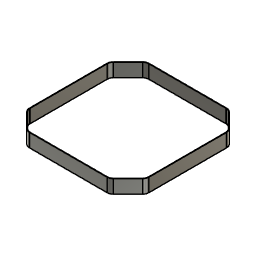
Drone Top Lid LED Face (Autodesk Fusion 360 design; units mm, degrees)
Autodesk Fusion 360 part; units mm, degrees
sketch "Sketch1" plane through (0, 0, 0) normal (0, 0, 1) x (1, 0, 0)
  line L0 (64.1079, 98.25) -> (-64.1079, 98.25)
  line L1 (-98.25, 64.1079) -> (-98.25, -64.1079)
  line L2 (-64.1079, -98.25) -> (64.1079, -98.25)
  line L3 (98.25, -64.1079) -> (98.25, 64.1079)
  line L4 (98.25, 98.25) -> (-98.25, -98.25) construction
  line L5 (-98.25, 98.25) -> (98.25, -98.25) construction
  line L6 (-95.3211, 71.1789) -> (-71.1789, 95.3211)
  arc A0 (-64.1079, 98.25) -> (-71.1789, 95.3211) centre (-64.1079, 88.25) ccw
  arc A1 (-95.3211, 71.1789) -> (-98.25, 64.1079) centre (-88.25, 64.1079) ccw
  line L7 (71.1789, 95.3211) -> (95.3211, 71.1789)
  line L8 (-95.3211, -71.1789) -> (-71.1789, -95.3211)
  line L9 (95.3211, -71.1789) -> (71.1789, -95.3211)
  arc A2 (71.1789, 95.3211) -> (64.1079, 98.25) centre (64.1079, 88.25) ccw
  arc A3 (98.25, 64.1079) -> (95.3211, 71.1789) centre (88.25, 64.1079) ccw
  arc A4 (95.3211, -71.1789) -> (98.25, -64.1079) centre (88.25, -64.1079) ccw
  arc A5 (64.1079, -98.25) -> (71.1789, -95.3211) centre (64.1079, -88.25) ccw
  arc A6 (-71.1789, -95.3211) -> (-64.1079, -98.25) centre (-64.1079, -88.25) ccw
  arc A7 (-98.25, -64.1079) -> (-95.3211, -71.1789) centre (-88.25, -64.1079) ccw
  point P0 (-98.25, 68.25)
  point P1 (-68.25, 98.25)
  point P2 (68.25, 98.25)
  point P3 (98.25, 68.25)
  point P4 (-98.25, -68.25)
  point P5 (-68.25, -98.25)
  point P6 (98.25, -68.25)
  point P7 (68.25, -98.25)
  dimension "d1" = 196.5
  dimension "d2" = 196.5
  dimension "d3" = 30
  dimension "d4" = 30
  dimension "d5" = 10
  dimension "d6" = 30
  dimension "d7" = 30
  dimension "d8" = 30
  dimension "d9" = 30
  dimension "d10" = 30
  dimension "d11" = 30
  dimension "d12" = 10
  constraint horizontal L0
  constraint perpendicular L0 L1
  constraint parallel L0 L2
  constraint parallel L1 L3
  constraint coincident L4 origin
  constraint coincident L5 origin
  constraint coincident L5.start L1
  constraint coincident L5.start L0
  constraint coincident P1 L6
  constraint coincident L0 P1
  constraint tangent L6 A0
  constraint tangent L0 A0
  constraint coincident P0 L6
  constraint coincident L1 P0
  constraint tangent L6 A1
  constraint tangent L1 A1
  constraint equal A0 A1
  constraint coincident L4.start L0
  constraint coincident L4.start L3
  constraint coincident L4.end L1
  constraint coincident L4.end L2
  constraint coincident L5.end L3
  constraint coincident L5.end L2
  constraint coincident P2 L7
  constraint coincident L0 P2
  constraint tangent L7 A2
  constraint tangent L0 A2
  constraint coincident P3 L7
  constraint coincident L3 P3
  constraint tangent L7 A3
  constraint tangent L3 A3
  constraint equal A2 A3
  constraint coincident P6 L9
  constraint coincident L3 P6
  constraint tangent L9 A4
  constraint tangent L3 A4
  constraint equal A2 A4
  constraint coincident P7 L9
  constraint coincident L2 P7
  constraint tangent L9 A5
  constraint tangent L2 A5
  constraint equal A2 A5
  constraint coincident P5 L8
  constraint coincident L2 P5
  constraint tangent L8 A6
  constraint tangent L2 A6
  constraint equal A2 A6
  constraint coincident P4 L8
  constraint coincident L1 P4
  constraint tangent L8 A7
  constraint tangent L1 A7
  constraint equal A2 A7
  measures "d1" distance of L4.end L5.end
  measures "d2" distance of L5.start L4.end
  measures "d3" distance of L5.start P0
  measures "d4" distance of L5.start P1
  measures "d5" radius of A0
  measures "d6" distance of L4.start P2
  measures "d7" distance of L4.start P3
  measures "d8" distance of L4.end P4
  measures "d9" distance of L4.end P5
  measures "d10" distance of L5.end P6
  measures "d11" distance of L5.end P7
  measures "d12" radius of A2
extrude "Extrude11" add sketch "Sketch1" along normal blind 22
sketch "Sketch21" plane through (0, 0, 0) normal (0, 0, 1) x (1, 0, 0)
  arc A0 (63.4579, -97.6) -> (70.5289, -94.6711) centre (63.4579, -87.6) ccw
  line L0 (97.6, -63.4579) -> (97.6, 63.4579)
  line L1 (94.6711, -70.5289) -> (70.5289, -94.6711)
  line L2 (-94.6711, 70.5289) -> (-70.5289, 94.6711)
  line L3 (-63.4579, -97.6) -> (63.4579, -97.6)
  line L4 (-97.6, 97.6) -> (97.6, -97.6) construction
  line L5 (-97.6, 63.4579) -> (-97.6, -63.4579)
  arc A1 (-94.6711, 70.5289) -> (-97.6, 63.4579) centre (-87.6, 63.4579) ccw
  arc A2 (97.6, 63.4579) -> (94.6711, 70.5289) centre (87.6, 63.4579) ccw
  arc A3 (-70.5289, -94.6711) -> (-63.4579, -97.6) centre (-63.4579, -87.6) ccw
  line L6 (70.5289, 94.6711) -> (94.6711, 70.5289)
  line L7 (97.6, 97.6) -> (-97.6, -97.6) construction
  line L8 (-94.6711, -70.5289) -> (-70.5289, -94.6711)
  arc A4 (-63.4579, 97.6) -> (-70.5289, 94.6711) centre (-63.4579, 87.6) ccw
  arc A5 (70.5289, 94.6711) -> (63.4579, 97.6) centre (63.4579, 87.6) ccw
  arc A6 (94.6711, -70.5289) -> (97.6, -63.4579) centre (87.6, -63.4579) ccw
  arc A7 (-97.6, -63.4579) -> (-94.6711, -70.5289) centre (-87.6, -63.4579) ccw
  line L9 (63.4579, 97.6) -> (-63.4579, 97.6)
  point P0 (-67.6, -97.6)
  point P1 (-97.6, -67.6)
  point P2 (67.6, -97.6)
  point P3 (-67.6, 97.6)
  point P4 (-97.6, 67.6)
  point P5 (97.6, 67.6)
  point P6 (97.6, -67.6)
  point P7 (67.6, 97.6)
  dimension "d179" = 195.2
  dimension "d180" = 195.2
  dimension "d181" = 30
  dimension "d182" = 30
  dimension "d183" = 10
  dimension "d184" = 30
  dimension "d185" = 30
  dimension "d186" = 30
  dimension "d187" = 30
  dimension "d188" = 30
  dimension "d189" = 30
  dimension "d190" = 10
  constraint horizontal L9
  constraint perpendicular L5 L9
  constraint parallel L3 L9
  constraint parallel L0 L5
  constraint coincident origin L7
  constraint coincident origin L4
  constraint coincident L4.start L5
  constraint coincident L4.start L9
  constraint coincident P3 L2
  constraint coincident P3 L9
  constraint tangent L2 A4
  constraint tangent A4 L9
  constraint coincident P4 L2
  constraint coincident P4 L5
  constraint tangent L2 A1
  constraint tangent L5 A1
  constraint equal A1 A4
  constraint coincident L7.start L9
  constraint coincident L7.start L0
  constraint coincident L7.end L5
  constraint coincident L7.end L3
  constraint coincident L4.end L0
  constraint coincident L4.end L3
  constraint coincident P7 L6
  constraint coincident P7 L9
  constraint tangent L6 A5
  constraint tangent A5 L9
  constraint coincident P5 L6
  constraint coincident P5 L0
  constraint tangent A2 L6
  constraint tangent L0 A2
  constraint equal A2 A5
  constraint coincident P6 L1
  constraint coincident P6 L0
  constraint tangent L1 A6
  constraint tangent L0 A6
  constraint equal A5 A6
  constraint coincident P2 L1
  constraint coincident P2 L3
  constraint tangent A0 L1
  constraint tangent A0 L3
  constraint equal A0 A5
  constraint coincident P0 L8
  constraint coincident P0 L3
  constraint tangent A3 L8
  constraint tangent L3 A3
  constraint equal A3 A5
  constraint coincident P1 L8
  constraint coincident P1 L5
  constraint tangent L8 A7
  constraint tangent L5 A7
  constraint equal A5 A7
  measures "d179" distance of L4.end L7.end
  measures "d180" distance of L4.start L7.end
  measures "d181" distance of P4 L4.start
  measures "d182" distance of P3 L4.start
  measures "d183" radius of A4
  measures "d184" distance of L7.start P7
  measures "d185" distance of P5 L7.start
  measures "d186" distance of P1 L7.end
  measures "d187" distance of P0 L7.end
  measures "d188" distance of L4.end P6
  measures "d189" distance of P2 L4.end
  measures "d190" radius of A5
extrude "Extrude19" cut sketch "Sketch21" along normal blind 30
equation "d4 = d3"
equation "d7 = d6"
equation "d9 = d8"
equation "d11 = d10"
equation "d182 = d3"
equation "d185 = d6"
equation "d187 = d8"
equation "d189 = d10"
